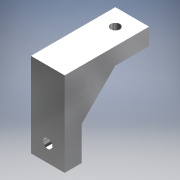
# Autodesk Inventor part: Standard Bracing
Saved by Autodesk Inventor 2019.4 (Build 234330000, 330)
## iProperties
Created: 2019-12-14
Part Number: Standard Bracing
Material: Aluminum 6061
Document SubType Name: Modeling
Designer: Mark
Mass: 59.4 g
Surface Area: 59.6569 cm^2
Volume: 22 cm^3
Density: 2.7 g/cm^3
Appearance: Aluminum - Flat
Author: Mark
Autodesk Inventor part; units mm, degrees
ref_plane "YZ Plane" through (0, 0, 0) normal (1, 0, 0) x (0, 1, 0)
ref_plane "XZ Plane" through (0, 0, 0) normal (0, 1, 0) x (-1, 0, 0)
ref_plane "XY Plane" through (0, 0, 0) normal (0, 0, 1) x (1, 0, 0)
sketch "Sketch1" plane through (0, 0, 0) normal (1, 0, 0) x (0, 1, 0)
  line L0 (0, 0) -> (20, 0)
  line L1 (20, 0) -> (20, -10)
  line L2 (20, -10) -> (0, -10)
  line L3 (0, -10) -> (0, 0)
  line L4 (20, -10) -> (50, -10)
  line L5 (50, -10) -> (50, 0)
  line L6 (50, 0) -> (20, 0)
  line L7 (20, 0) -> (20, -10)
  line L8 (50, 0) -> (40, 0)
  line L9 (40, 0) -> (40, -50)
  line L10 (40, -50) -> (50, -50)
  line L11 (50, -50) -> (50, 0)
  line L12 (40, -50) -> (50, -50)
  line L13 (50, -50) -> (50, -30)
  line L14 (50, -30) -> (40, -30)
  line L15 (40, -30) -> (40, -50)
  line L16 (20, -10) -> (40, -30)
  line L17 (40, -10) -> (20, -10)
  line L18 (40, -10) -> (40, -30)
  dimension "d0" = 20
  dimension "d1" = 10
  dimension "d2" = 30
  dimension "d3" = 10
  dimension "d4" = 10
  dimension "d5" = 50
  dimension "d6" = 10
  dimension "d7" = 20
  constraints: 38 end point, 9 equal length, 4 horizontal, 4 perpendicular, 2 point on line
  measures "d0" distance of L1.end L2.end
  measures "d1" distance of L0.end L1.end
  measures "d2" distance of L6.end L5.end
  measures "d3" distance of L5.end L4.end
  measures "d4" distance of L10.end L9.end
  measures "d5" distance of L9.end L8.end
  measures "d6" distance of L14.end L13.end
  measures "d7" distance of L13.end L12.end
extrude "Extrusion1" add sketch "Sketch1" along normal blind 20
sketch "Sketch2" plane through (0, 50, 0) normal (0, 1, 0) x (1, 0, 0)
  circle A0 centre (10, 40) radius 2.75
  line L0 (20, 50) -> (20, 0) projected
  line L1 (0, 50) -> (20, 50) projected
  point P0 (0, 0)
  dimension "d10" = 5.5
  dimension "d11" = 10
  dimension "d12" = 10
  constraints: 1 centre point
  measures "d10" diameter of A0
  measures "d11" distance from line of A0.centre L0
  measures "d12" distance from line of L1 A0.centre
extrude "Extrusion2" cut sketch "Sketch2" against normal blind 20
sketch "Sketch3" plane through (0, 0, 0) normal (0, 0, 1) x (1, 0, 0)
  circle A0 centre (10, 10) radius 2.75
  line L0 (0, 0) -> (20, 0) projected
  line L1 (20, 50) -> (20, 0) projected
  dimension "d15" = 5.5
  dimension "d16" = 10
  dimension "d17" = 10
  constraints: 1 centre point
  measures "d15" diameter of A0
  measures "d16" distance from line of A0.centre L0
  measures "d17" distance from line of L1 A0.centre
extrude "Extrusion3" cut sketch "Sketch3" against normal blind 20
body "Solid1"
